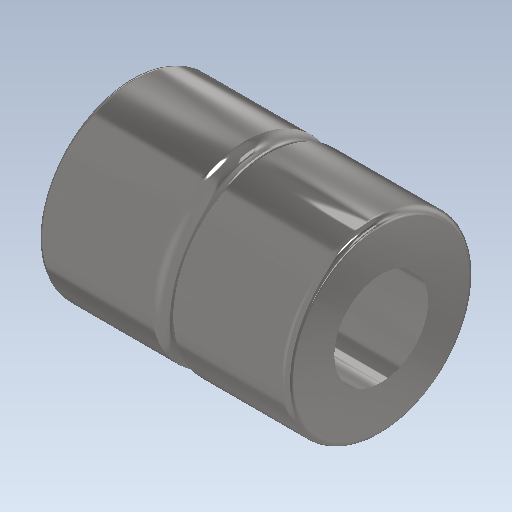
# Autodesk Inventor part: LMUT6
Saved by Autodesk Inventor 2021 (Build 250183000, 183)
## iProperties
Category: PARTsolutions
Company: MISUMI
Part Number: LMUT6
Material: 鉄、鋳鉄
Catalog Web Link: www.cadenas.de
Description: LMUT, SLMUT-Linear Bushings - Short Type
Vendor: MISUMI
Document SubType Name: Modeling
Designer: partserver
Manufacturer: MISUMI
Mass: 9.60748 g
Surface Area: 10.6549 cm^2
Volume: 1.3437 cm^3
Density: 7.15 g/cm^3
Appearance: 鋼 - つや出し
PSOL_IDENT_0: {$CADENAS_DATA\23d-libs\misumi\metric\04_linear_bushings\lmut.prj},167 {VTYP=3D},{NB=LMUT6},{LINA=LM
PSOL_IDENT_1: UT6},{NN=LMUT, SLMUT},{DATE=09.09.2019 15:26:51},{GEOMDATE=27.08.2015 04:41:47},{VERSION=},{LINEID=4
PSOL_IDENT_2: 0},{WBVAR=MATOC,GREASE},{WBNUMERIC=}  {NB=LMUT6},{LINA=LMUT6},{KT=DUMMY},{PN=LMUT6},{MATOC=1},{HARDO
PSOL_IDENT_3: C=58HRC~},{MATB=SUJ2(52100 Bearing Steel)(1.3505_100Cr6)},{MATR=Resin (Duracone M90, or Equivalent)}
PSOL_IDENT_4: ,{OT=-20~80},{AC=Adhesive},{MATA=Nitrile Rubber (-20~120 deg Celsius)},{GREASE=},{TYPE=LMUT},{DDRR=6
PSOL_IDENT_5: },{DDRRTOL=0/-0.009},{D=12},{DTOL=0/-0.011},{L=16},{LTOL=0/-0.2},{R=1.0},{FF=0.3},{RR=0.4},{ESS=0.01
PSOL_IDENT_6: 2},{BR=4},{CD=113},{CO=155},{MASS=6.6}
NN: LMUT, SLMUT
NT: Linear Bushings - Short Type
NB: LMUT6
NBSYN: $PN.
LINA: LMUT6
PN: LMUT6
MATOC: 52100 Bearing Steel
HARDOC: 58HRC~
MATB: 52100 Bearing Steel
MATR: Resin (Duracone M90, or Equivalent)
OT: -20~80
AC: Adhesive
MATA: Nitrile Rubber (-20~120 deg Celsius)
GREASE: Normal (For general Use)
DDRR: 6
DDRRTOL: 0/-0.009
D: 12
DTOL: 0/-0.011
L: 16
LTOL: 0/-0.2
R: 1
FF: 0.3
RR: 0.4
ESS: 0.012
BR: 4
CD: 113
CO: 155
MASS: 6.6
SUPPLIER: MISUMI
ARTICLENO: LMUT6
BOMINFO: LMUT6
CREATOR: CADENAS GmbH
Title: LMUT6
Author: Cadenas PARTsolutions
Comments: Linear Bushings - Short Type
Autodesk Inventor part; units mm, degrees
ref_plane "YZ Plane" through (0, 0, 0) normal (1, 0, 0) x (0, 1, 0)
ref_plane "XZ Plane" through (0, 0, 0) normal (0, 1, 0) x (-1, 0, 0)
ref_plane "XY Plane" through (0, 0, 0) normal (0, 0, 1) x (1, 0, 0)
sketch "Sketch_1" plane through (0, 0, 0) normal (0, 0, 1) x (1, 0, 0)
  line L0 (16, 0) -> (0, 0)
  line L1 (0, 0) -> (0, 5.6)
  arc A0 (0.4, 6) -> (0, 5.6) centre (0.4, 5.6) ccw
  line L2 (0.4, 6) -> (7.2859, 6)
  arc A1 (7.2859, 6) -> (8.7141, 6) centre (8, 6.7) ccw
  line L3 (8.7141, 6) -> (15.6, 6)
  arc A2 (16, 5.6) -> (15.6, 6) centre (15.6, 5.6) ccw
  line L4 (16, 5.6) -> (16, 0)
  line L5 (16, 0) -> (0, 0)
  constraints: 12 end point, 6 point on circle, 3 centre point
revolve "Revolution1" add sketch "Sketch_1" angle 360 about axis through (16, 0, 0) along (1, 0, 0)
sketch "Sketch2" plane through (16, 0, 0) normal (1, 0, 0) x (0, 0, -1)
  point P0 (0, 0)
hole "Hole1" at (16, 0, 0) direction (-1, 0, 0) diameter 6 depth 16
body "Solid1"
